Autodesk Inventor part; units mm, degrees
(part 2 of 2)
  line L452 (2.0688, 5.6455) -> (1.7172, 5.9716)
  line L453 (1.7172, 5.9716) -> (1.2814, 5.6264)
  line L454 (1.2814, 5.1401) -> (1.2814, 5.5243)
  line L455 (1.2814, 5.5243) -> (1.3618, 5.5243)
  line L456 (1.3618, 5.5243) -> (1.3618, 5.3813)
  line L457 (1.3618, 5.3813) -> (1.8895, 5.3813)
  line L458 (1.8895, 5.3813) -> (1.8895, 5.5243)
  line L459 (1.8895, 5.5243) -> (1.9616, 5.5243)
  spline S169 degree 2 poles (1.9616, 5.5243) (1.9616, 5.4432) (2.0075, 5.3667) (2.0713, 5.3616) knots 0 0 0 1 2 2 2
  line L460 (2.0713, 5.3616) -> (2.0713, 5.2799)
  line L461 (2.0713, 5.2799) -> (1.3618, 5.2799)
  line L462 (1.3618, 5.2799) -> (1.3618, 5.1401)
  line L463 (1.3618, 5.1401) -> (1.2814, 5.1401)
  line L464 (1.5519, 4.4887) -> (1.5519, 4.5825)
  line L465 (1.5519, 4.5825) -> (1.2814, 4.5825)
  line L466 (1.2814, 4.5825) -> (1.2814, 4.6839)
  line L467 (1.2814, 4.6839) -> (1.5519, 4.6839)
  line L468 (1.5519, 4.6839) -> (1.5519, 5.0317)
  line L469 (1.5519, 5.0317) -> (1.6629, 5.0317)
  line L470 (1.6629, 5.0317) -> (2.0688, 4.6794)
  line L471 (2.0688, 4.6794) -> (2.0688, 4.5825)
  line L472 (2.0688, 4.5825) -> (1.6368, 4.5825)
  line L473 (1.6368, 4.5825) -> (1.6368, 4.4887)
  line L474 (1.6368, 4.4887) -> (1.5519, 4.4887)
  line L475 (1.6368, 4.6839) -> (1.9443, 4.6839)
  line L476 (1.9443, 4.6839) -> (1.6368, 4.9487)
  line L477 (1.6368, 4.9487) -> (1.6368, 4.6839)
  point P0 (0, 0)
  dimension "d0" = 53.34
  dimension "d1" = 66.04
  dimension "d2" = 66.04
  dimension "d3" = 2.032
  dimension "d4" = 12.7
  dimension "d5" = 2.286
  dimension "d6" = 33.401
  dimension "d23" = 0.4572
  dimension "d24" = 1.651
  dimension "d25" = 0.4572
  dimension "d26" = 1.651
  dimension "d27" = 0.4572
  dimension "d28" = 0.4572
  dimension "d29" = 0.4572
  dimension "d30" = 0.6397
  dimension "d31" = 1.651
  constraints: 11 collinear, 9 coincident, 20 other
  measures "d23" distance between parallel lines of L35 L38
  measures "d24" distance between parallel lines of L36 L41
  measures "d25" distance between parallel lines of L0 L42
  measures "d26" distance between parallel lines of L13 L49
  measures "d27" distance between parallel lines of L16 L46
  measures "d28" distance between parallel lines of L66 L10
  measures "d29" distance between parallel lines of L6 L62
  measures "d30" distance between parallel lines of L2 L58
  measures "d31" distance between parallel lines of L29 L53
extrude "DET1" add sketch "Sketch3" along normal blind 0.254 contours S0 L78 L79 S1 S2 S3 S4 S5 S6 S7 S8 L80 L81 S9 S10 S11 S12 S13 S14 S15 | L82 L83 L84 L85 L86 L87 L88 L89 L90 L91 L92 L93 | L94 L95 L96 L97 L98 L99 S16 L100 L101 L102 L103 | L104 L105 L106 L107 L108 L109 L110 L111 L112 L113 L114 | S17 L118 L119 S18 S19 S20 S21 S22 S23 S24 S25 L120 L121 S26 S27 S28 S29 S30 S31 S32 | L122 L123 L124 L125 L126 L127 L128 L129 L130 L131 L132 L133 | L134 L135 L136 L137 L138 L139 S33 L140 L141 L142 L143 | L144 L145 L146 L147 L148 L149 L150 L151 L152 L153 L154 | S34 L158 L159 S35 S36 S37 S38 S39 S40 S41 S42 L160 L161 S43 S44 S45 S46 S47 S48 S49 | L162 L163 L164 L165 L166 L167 L168 L169 L170 L171 L172 L173 | L174 L175 L176 L177 L178 L179 S50 L180 L181 L182 L183 | L184 L185 L186 L187 L188 L189 L190 L191 L192 L193 L194 | S51 L198 L199 S52 S53 S54 S55 S56 S57 S58 S59 L200 L201 S60 S61 S62 S63 S64 S65 S66 | L202 L203 L204 L205 L206 L207 L208 L209 L210 L211 L212 L213 | L214 L215 L216 L217 L218 L219 S67 L220 L221 L222 L223 | L224 L225 L226 L227 L228 L229 L230 L231 L232 L233 L234 | S68 L238 L239 S69 S70 S71 S72 S73 S74 S75 S76 L240 L241 S77 S78 S79 S80 S81 S82 S83 | L242 L243 L244 L245 L246 L247 L248 L249 L250 L251 L252 L253 | L254 L255 L256 L257 L258 L259 S84 L260 L261 L262 L263 | L264 L265 L266 L267 L268 L269 L270 L271 L272 L273 L274 | S85 L278 L279 S86 S87 S88 S89 S90 S91 S92 S93 L280 L281 S94 S95 S96 S97 S98 S99 S100 | L282 L283 L284 L285 L286 L287 L288 L289 L290 L291 L292 L293 | L294 L295 L296 L297 L298 L299 S101 L300 L301 L302 L303 | L304 L305 L306 L307 L308 L309 L310 L311 L312 L313 L314 | S102 L318 L319 S103 S104 S105 S106 S107 S108 S109 S110 L320 L321 S111 S112 S113 S114 S115 S116 S117 | L322 L323 L324 L325 L326 L327 L328 L329 L330 L331 L332 L333 | L334 L335 L336 L337 L338 L339 S118 L340 L341 L342 L343 | L344 L345 L346 L347 L348 L349 L350 L351 L352 L353 L354 | S119 L358 L359 S120 S121 S122 S123 S124 S125 S126 S127 L360 L361 S128 S129 S130 S131 S132 S133 S134 | L362 L363 L364 L365 L366 L367 L368 L369 L370 L371 L372 L373 | L374 L375 L376 L377 L378 L379 S135 L380 L381 L382 L383 | L384 L385 L386 L387 L388 L389 L390 L391 L392 L393 L394 | S136 L398 L399 S137 S138 S139 S140 S141 S142 S143 S144 L400 L401 S145 S146 S147 S148 S149 S150 S151 | L402 L403 L404 L405 L406 L407 L408 L409 L410 L411 L412 L413 | L414 L415 L416 L417 L418 L419 S152 L420 L421 L422 L423 | L424 L425 L426 L427 L428 L429 L430 L431 L432 L433 L434 | S153 L438 L439 S154 S155 S156 S157 S158 S159 S160 S161 L440 L441 S162 S163 S164 S165 S166 S167 S168 | L442 L443 L444 L445 L446 L447 L448 L449 L450 L451 L452 L453 | L454 L455 L456 L457 L458 L459 S169 L460 L461 L462 L463 | L464 L465 L466 L467 L468 L469 L470 L471 L472 L473 L474
sketch "Sketch4" plane through (0, 1.524, 0) normal (0, 1, 0) x (1, 0, 0)
  line L0 (-26.67, 33.02) -> (-26.67, -33.02) projected
  line L1 (13.97, -33.02) -> (26.67, -33.02) projected
  line L2 (26.67, -33.02) -> (26.67, 33.02) projected
  line L3 (25.4, -31.75) -> (22.86, -31.75)
  line L4 (22.86, -31.75) -> (22.86, -11.43)
  line L5 (22.86, -11.43) -> (25.4, -11.43)
  line L6 (25.4, -11.43) -> (25.4, -31.75)
  line L7 (24.13, -31.75) -> (24.13, -11.43) construction
  line L8 (22.86, -10.287) -> (25.4, -10.287)
  line L9 (25.4, -10.287) -> (25.4, 15.113)
  line L10 (25.4, 15.113) -> (22.86, 15.113)
  line L11 (22.86, 15.113) -> (22.86, -10.287)
  line L12 (23.749, 14.224) -> (24.511, 14.224)
  line L13 (24.511, 14.224) -> (24.511, 13.462)
  line L14 (24.511, 13.462) -> (23.749, 13.462)
  line L15 (23.749, 13.462) -> (23.749, 14.224)
  line L16 (24.511, 13.462) -> (23.749, 14.224) construction
  line L17 (23.749, 13.462) -> (24.511, 14.224) construction
  line L18 (23.749, 11.684) -> (24.511, 11.684)
  line L19 (24.511, 11.684) -> (24.511, 10.922)
  line L20 (24.511, 10.922) -> (23.749, 10.922)
  line L21 (23.749, 10.922) -> (23.749, 11.684)
  line L22 (23.749, 9.144) -> (24.511, 9.144)
  line L23 (24.511, 9.144) -> (24.511, 8.382)
  line L24 (24.511, 8.382) -> (23.749, 8.382)
  line L25 (23.749, 8.382) -> (23.749, 9.144)
  line L26 (23.749, 6.604) -> (24.511, 6.604)
  line L27 (24.511, 6.604) -> (24.511, 5.842)
  line L28 (24.511, 5.842) -> (23.749, 5.842)
  line L29 (23.749, 5.842) -> (23.749, 6.604)
  line L30 (23.749, 4.064) -> (24.511, 4.064)
  line L31 (24.511, 4.064) -> (24.511, 3.302)
  line L32 (24.511, 3.302) -> (23.749, 3.302)
  line L33 (23.749, 3.302) -> (23.749, 4.064)
  line L34 (23.749, 1.524) -> (24.511, 1.524)
  line L35 (24.511, 1.524) -> (24.511, 0.762)
  line L36 (24.511, 0.762) -> (23.749, 0.762)
  line L37 (23.749, 0.762) -> (23.749, 1.524)
  line L38 (23.749, -1.016) -> (24.511, -1.016)
  line L39 (24.511, -1.016) -> (24.511, -1.778)
  line L40 (24.511, -1.778) -> (23.749, -1.778)
  line L41 (23.749, -1.778) -> (23.749, -1.016)
  line L42 (23.749, -3.556) -> (24.511, -3.556)
  line L43 (24.511, -3.556) -> (24.511, -4.318)
  line L44 (24.511, -4.318) -> (23.749, -4.318)
  line L45 (23.749, -4.318) -> (23.749, -3.556)
  line L46 (23.749, -6.096) -> (24.511, -6.096)
  line L47 (24.511, -6.096) -> (24.511, -6.858)
  line L48 (24.511, -6.858) -> (23.749, -6.858)
  line L49 (23.749, -6.858) -> (23.749, -6.096)
  line L50 (23.749, -8.636) -> (24.511, -8.636)
  line L51 (24.511, -8.636) -> (24.511, -9.398)
  line L52 (24.511, -9.398) -> (23.749, -9.398)
  line L53 (23.749, -9.398) -> (23.749, -8.636)
  line L54 (23.749, -12.319) -> (24.511, -12.319)
  line L55 (24.511, -12.319) -> (24.511, -13.081)
  line L56 (24.511, -13.081) -> (23.749, -13.081)
  line L57 (23.749, -13.081) -> (23.749, -12.319)
  line L58 (23.749, -12.319) -> (24.511, -13.081) construction
  line L59 (24.511, -12.319) -> (23.749, -13.081) construction
  line L60 (23.749, -14.859) -> (24.511, -14.859)
  line L61 (24.511, -14.859) -> (24.511, -15.621)
  line L62 (24.511, -15.621) -> (23.749, -15.621)
  line L63 (23.749, -15.621) -> (23.749, -14.859)
  line L64 (23.749, -17.399) -> (24.511, -17.399)
  line L65 (24.511, -17.399) -> (24.511, -18.161)
  line L66 (24.511, -18.161) -> (23.749, -18.161)
  line L67 (23.749, -18.161) -> (23.749, -17.399)
  line L68 (23.749, -19.939) -> (24.511, -19.939)
  line L69 (24.511, -19.939) -> (24.511, -20.701)
  line L70 (24.511, -20.701) -> (23.749, -20.701)
  line L71 (23.749, -20.701) -> (23.749, -19.939)
  line L72 (23.749, -22.479) -> (24.511, -22.479)
  line L73 (24.511, -22.479) -> (24.511, -23.241)
  line L74 (24.511, -23.241) -> (23.749, -23.241)
  line L75 (23.749, -23.241) -> (23.749, -22.479)
  line L76 (23.749, -25.019) -> (24.511, -25.019)
  line L77 (24.511, -25.019) -> (24.511, -25.781)
  line L78 (24.511, -25.781) -> (23.749, -25.781)
  line L79 (23.749, -25.781) -> (23.749, -25.019)
  line L80 (23.749, -27.559) -> (24.511, -27.559)
  line L81 (24.511, -27.559) -> (24.511, -28.321)
  line L82 (24.511, -28.321) -> (23.749, -28.321)
  line L83 (23.749, -28.321) -> (23.749, -27.559)
  line L84 (23.749, -30.099) -> (24.511, -30.099)
  line L85 (24.511, -30.099) -> (24.511, -30.861)
  line L86 (24.511, -30.861) -> (23.749, -30.861)
  line L87 (23.749, -30.861) -> (23.749, -30.099)
  line L88 (-21.59, -31.75) -> (-24.13, -31.75)
  line L89 (-24.13, -31.75) -> (-24.13, -16.51)
  line L90 (-24.13, -16.51) -> (-21.59, -16.51)
  line L91 (-21.59, -16.51) -> (-21.59, -31.75)
  line L92 (-22.479, -17.399) -> (-23.241, -17.399)
  line L93 (-23.241, -17.399) -> (-23.241, -18.161)
  line L94 (-23.241, -18.161) -> (-22.479, -18.161)
  line L95 (-22.479, -18.161) -> (-22.479, -17.399)
  line L96 (-22.479, -18.161) -> (-23.241, -17.399) construction
  line L97 (-22.479, -17.399) -> (-23.241, -18.161) construction
  line L98 (-22.479, -19.939) -> (-23.241, -19.939)
  line L99 (-23.241, -19.939) -> (-23.241, -20.701)
  line L100 (-23.241, -20.701) -> (-22.479, -20.701)
  line L101 (-22.479, -20.701) -> (-22.479, -19.939)
  line L102 (-22.479, -22.479) -> (-23.241, -22.479)
  line L103 (-23.241, -22.479) -> (-23.241, -23.241)
  line L104 (-23.241, -23.241) -> (-22.479, -23.241)
  line L105 (-22.479, -23.241) -> (-22.479, -22.479)
  line L106 (-22.479, -25.019) -> (-23.241, -25.019)
  line L107 (-23.241, -25.019) -> (-23.241, -25.781)
  line L108 (-23.241, -25.781) -> (-22.479, -25.781)
  line L109 (-22.479, -25.781) -> (-22.479, -25.019)
  line L110 (-22.479, -27.559) -> (-23.241, -27.559)
  line L111 (-23.241, -27.559) -> (-23.241, -28.321)
  line L112 (-23.241, -28.321) -> (-22.479, -28.321)
  line L113 (-22.479, -28.321) -> (-22.479, -27.559)
  line L114 (-22.479, -30.099) -> (-23.241, -30.099)
  line L115 (-23.241, -30.099) -> (-23.241, -30.861)
  line L116 (-23.241, -30.861) -> (-22.479, -30.861)
  line L117 (-22.479, -30.861) -> (-22.479, -30.099)
  line L118 (-24.13, -15.367) -> (-21.59, -15.367)
  line L119 (-21.59, -15.367) -> (-21.59, 4.953)
  line L120 (-21.59, 4.953) -> (-24.13, 4.953)
  line L121 (-24.13, 4.953) -> (-24.13, -15.367)
  line L122 (-23.241, 4.064) -> (-22.479, 4.064)
  line L123 (-22.479, 4.064) -> (-22.479, 3.302)
  line L124 (-22.479, 3.302) -> (-23.241, 3.302)
  line L125 (-23.241, 3.302) -> (-23.241, 4.064)
  line L126 (-23.241, 1.524) -> (-22.479, 1.524)
  line L127 (-22.479, 1.524) -> (-22.479, 0.762)
  line L128 (-22.479, 0.762) -> (-23.241, 0.762)
  line L129 (-23.241, 0.762) -> (-23.241, 1.524)
  line L130 (-23.241, -1.016) -> (-22.479, -1.016)
  line L131 (-22.479, -1.016) -> (-22.479, -1.778)
  line L132 (-22.479, -1.778) -> (-23.241, -1.778)
  line L133 (-23.241, -1.778) -> (-23.241, -1.016)
  line L134 (-23.241, -3.556) -> (-22.479, -3.556)
  line L135 (-22.479, -3.556) -> (-22.479, -4.318)
  line L136 (-22.479, -4.318) -> (-23.241, -4.318)
  line L137 (-23.241, -4.318) -> (-23.241, -3.556)
  line L138 (-23.241, -6.096) -> (-22.479, -6.096)
  line L139 (-22.479, -6.096) -> (-22.479, -6.858)
  line L140 (-22.479, -6.858) -> (-23.241, -6.858)
  line L141 (-23.241, -6.858) -> (-23.241, -6.096)
  line L142 (-23.241, -8.636) -> (-22.479, -8.636)
  line L143 (-22.479, -8.636) -> (-22.479, -9.398)
  line L144 (-22.479, -9.398) -> (-23.241, -9.398)
  line L145 (-23.241, -9.398) -> (-23.241, -8.636)
  line L146 (-23.241, -11.176) -> (-22.479, -11.176)
  line L147 (-22.479, -11.176) -> (-22.479, -11.938)
  line L148 (-22.479, -11.938) -> (-23.241, -11.938)
  line L149 (-23.241, -11.938) -> (-23.241, -11.176)
  line L150 (-23.241, -13.716) -> (-22.479, -13.716)
  line L151 (-22.479, -13.716) -> (-22.479, -14.478)
  line L152 (-22.479, -14.478) -> (-23.241, -14.478)
  line L153 (-23.241, -14.478) -> (-23.241, -13.716)
  point P0 (0, 0)
  point P1 (24.13, 13.843)
  point P2 (24.13, -12.7)
  point P3 (-22.86, -17.78)
  dimension "d34" = 2.54
  dimension "d36" = 20.32
  dimension "d37" = 1.27
  dimension "d38" = 1.27
  dimension "d39" = 25.4
  dimension "d40" = 1.143
  dimension "d42" = 0.762
  dimension "d44" = 1.27
  dimension "d46" = 1.27
  dimension "d49" = 2.54
  dimension "d54" = 1.27
  dimension "d57" = 2.54
  dimension "d62" = 0.889
  dimension "d63" = 0.889
  dimension "d64" = 2.54
  dimension "d65" = 15.24
  dimension "d66" = 0.762
  dimension "d68" = 0.889
  dimension "d69" = 1.27
  dimension "d72" = 2.54
  dimension "d77" = 20.32
  dimension "d78" = 1.143
  dimension "d79" = 0.762
  dimension "d81" = 0.889
  dimension "d84" = 2.54
  constraints: 302 end point, 16 parallel, 10 perpendicular, 8 horizontal, 7 equal length, 6 collinear, 5 midpoint, 4 vertical, 224 other
  measures "d34" distance between parallel lines of L6 L4
  measures "d36" distance of L5.end L3.start
  measures "d37" distance between parallel lines of L6 L2
  measures "d38" distance between parallel lines of L1 L3
  measures "d39" distance of L8.end L9.end
  measures "d40" distance between parallel lines of L5 L8
  measures "d42" distance of L12.end L13.end
  measures "d44" distance from line of L11 point (24.13, 13.843)
  measures "d46" distance from line of L10 point (24.13, 13.843)
  measures "d49" distance of L12.end L19.start
  measures "d54" distance from line of L5 point (24.13, -12.7)
  measures "d57" distance of L56.end L63.start
  measures "d62" distance between parallel lines of L3 L86
  measures "d63" distance between parallel lines of L8 L52
  measures "d64" distance between parallel lines of L0 L89
  measures "d65" distance of L88.end L89.end
  measures "d66" distance of L94.end L93.end
  measures "d68" distance between parallel lines of L89 L93
  measures "d69" distance from line of L90 point (-22.86, -17.78)
  measures "d72" distance of L94.end L101.start
  measures "d77" distance of L120.end L118.start
  measures "d78" distance between parallel lines of L90 L118
  measures "d79" distance of L122.start L122.end
  measures "d81" distance between parallel lines of L120 L122
  measures "d84" distance of L123.end L128.start
extrude "Extrusion4" add sketch "Sketch4" along normal blind 8.636
sketch "Sketch5" plane through (0, 1.524, 0) normal (0, 1, 0) x (1, 0, 0)
  line L0 (-22.479, 3.302) -> (-22.479, 4.064) projected
  line L1 (-22.479, 4.064) -> (-23.241, 4.064) projected
  line L2 (-23.241, 4.064) -> (-23.241, 3.302) projected
  line L3 (-23.241, 3.302) -> (-22.479, 3.302) projected
  line L4 (-23.241, 0.762) -> (-22.479, 0.762) projected
  line L5 (-22.479, 0.762) -> (-22.479, 1.524) projected
  line L6 (-22.479, 1.524) -> (-23.241, 1.524) projected
  line L7 (-23.241, 1.524) -> (-23.241, 0.762) projected
  line L8 (-23.241, -1.778) -> (-22.479, -1.778) projected
  line L9 (-22.479, -1.778) -> (-22.479, -1.016) projected
  line L10 (-22.479, -1.016) -> (-23.241, -1.016) projected
  line L11 (-23.241, -1.016) -> (-23.241, -1.778) projected
  line L12 (-23.241, -4.318) -> (-22.479, -4.318) projected
  line L13 (-22.479, -4.318) -> (-22.479, -3.556) projected
  line L14 (-22.479, -3.556) -> (-23.241, -3.556) projected
  line L15 (-23.241, -3.556) -> (-23.241, -4.318) projected
  line L16 (-23.241, -6.858) -> (-22.479, -6.858) projected
  line L17 (-22.479, -6.858) -> (-22.479, -6.096) projected
  line L18 (-22.479, -6.096) -> (-23.241, -6.096) projected
  line L19 (-23.241, -6.096) -> (-23.241, -6.858) projected
  line L20 (-23.241, -9.398) -> (-22.479, -9.398) projected
  line L21 (-22.479, -9.398) -> (-22.479, -8.636) projected
  line L22 (-22.479, -8.636) -> (-23.241, -8.636) projected
  line L23 (-23.241, -8.636) -> (-23.241, -9.398) projected
  line L24 (-23.241, -11.938) -> (-22.479, -11.938) projected
  line L25 (-22.479, -11.938) -> (-22.479, -11.176) projected
  line L26 (-22.479, -11.176) -> (-23.241, -11.176) projected
  line L27 (-23.241, -11.176) -> (-23.241, -11.938) projected
  line L28 (-23.241, -14.478) -> (-22.479, -14.478) projected
  line L29 (-22.479, -14.478) -> (-22.479, -13.716) projected
  line L30 (-22.479, -13.716) -> (-23.241, -13.716) projected
  line L31 (-23.241, -13.716) -> (-23.241, -14.478) projected
  line L32 (-22.479, -18.161) -> (-22.479, -17.399) projected
  line L33 (-22.479, -17.399) -> (-23.241, -17.399) projected
  line L34 (-23.241, -17.399) -> (-23.241, -18.161) projected
  line L35 (-23.241, -18.161) -> (-22.479, -18.161) projected
  line L36 (-23.241, -19.939) -> (-23.241, -20.701) projected
  line L37 (-23.241, -20.701) -> (-22.479, -20.701) projected
  line L38 (-22.479, -20.701) -> (-22.479, -19.939) projected
  line L39 (-22.479, -19.939) -> (-23.241, -19.939) projected
  line L40 (-23.241, -22.479) -> (-23.241, -23.241) projected
  line L41 (-23.241, -23.241) -> (-22.479, -23.241) projected
  line L42 (-22.479, -23.241) -> (-22.479, -22.479) projected
  line L43 (-22.479, -22.479) -> (-23.241, -22.479) projected
  line L44 (-23.241, -25.019) -> (-23.241, -25.781) projected
  line L45 (-23.241, -25.781) -> (-22.479, -25.781) projected
  line L46 (-22.479, -25.781) -> (-22.479, -25.019) projected
  line L47 (-22.479, -25.019) -> (-23.241, -25.019) projected
  line L48 (-23.241, -27.559) -> (-23.241, -28.321) projected
  line L49 (-23.241, -28.321) -> (-22.479, -28.321) projected
  line L50 (-22.479, -28.321) -> (-22.479, -27.559) projected
  line L51 (-22.479, -27.559) -> (-23.241, -27.559) projected
  line L52 (-23.241, -30.099) -> (-23.241, -30.861) projected
  line L53 (-23.241, -30.861) -> (-22.479, -30.861) projected
  line L54 (-22.479, -30.861) -> (-22.479, -30.099) projected
  line L55 (-22.479, -30.099) -> (-23.241, -30.099) projected
  line L56 (24.511, 13.462) -> (24.511, 14.224) projected
  line L57 (24.511, 14.224) -> (23.749, 14.224) projected
  line L58 (23.749, 14.224) -> (23.749, 13.462) projected
  line L59 (23.749, 13.462) -> (24.511, 13.462) projected
  line L60 (24.511, 10.922) -> (24.511, 11.684) projected
  line L61 (24.511, 11.684) -> (23.749, 11.684) projected
  line L62 (23.749, 11.684) -> (23.749, 10.922) projected
  line L63 (23.749, 10.922) -> (24.511, 10.922) projected
  line L64 (24.511, 8.382) -> (24.511, 9.144) projected
  line L65 (24.511, 9.144) -> (23.749, 9.144) projected
  line L66 (23.749, 9.144) -> (23.749, 8.382) projected
  line L67 (23.749, 8.382) -> (24.511, 8.382) projected
  line L68 (24.511, 5.842) -> (24.511, 6.604) projected
  line L69 (24.511, 6.604) -> (23.749, 6.604) projected
  line L70 (23.749, 6.604) -> (23.749, 5.842) projected
  line L71 (23.749, 5.842) -> (24.511, 5.842) projected
  line L72 (24.511, 3.302) -> (24.511, 4.064) projected
  line L73 (24.511, 4.064) -> (23.749, 4.064) projected
  line L74 (23.749, 4.064) -> (23.749, 3.302) projected
  line L75 (23.749, 3.302) -> (24.511, 3.302) projected
  line L76 (24.511, 0.762) -> (24.511, 1.524) projected
  line L77 (24.511, 1.524) -> (23.749, 1.524) projected
  line L78 (23.749, 1.524) -> (23.749, 0.762) projected
  line L79 (23.749, 0.762) -> (24.511, 0.762) projected
  line L80 (24.511, -1.778) -> (24.511, -1.016) projected
  line L81 (24.511, -1.016) -> (23.749, -1.016) projected
  line L82 (23.749, -1.016) -> (23.749, -1.778) projected
  line L83 (23.749, -1.778) -> (24.511, -1.778) projected
  line L84 (24.511, -4.318) -> (24.511, -3.556) projected
  line L85 (24.511, -3.556) -> (23.749, -3.556) projected
  line L86 (23.749, -3.556) -> (23.749, -4.318) projected
  line L87 (23.749, -4.318) -> (24.511, -4.318) projected
  line L88 (24.511, -6.858) -> (24.511, -6.096) projected
  line L89 (24.511, -6.096) -> (23.749, -6.096) projected
  line L90 (23.749, -6.096) -> (23.749, -6.858) projected
  line L91 (23.749, -6.858) -> (24.511, -6.858) projected
  line L92 (24.511, -9.398) -> (24.511, -8.636) projected
  line L93 (24.511, -8.636) -> (23.749, -8.636) projected
  line L94 (23.749, -8.636) -> (23.749, -9.398) projected
  line L95 (23.749, -9.398) -> (24.511, -9.398) projected
  line L96 (24.511, -13.081) -> (24.511, -12.319) projected
  line L97 (24.511, -12.319) -> (23.749, -12.319) projected
  line L98 (23.749, -12.319) -> (23.749, -13.081) projected
  line L99 (23.749, -13.081) -> (24.511, -13.081) projected
  line L100 (23.749, -14.859) -> (23.749, -15.621) projected
  line L101 (23.749, -15.621) -> (24.511, -15.621) projected
  line L102 (24.511, -15.621) -> (24.511, -14.859) projected
  line L103 (24.511, -14.859) -> (23.749, -14.859) projected
  line L104 (23.749, -17.399) -> (23.749, -18.161) projected
  line L105 (23.749, -18.161) -> (24.511, -18.161) projected
  line L106 (24.511, -18.161) -> (24.511, -17.399) projected
  line L107 (24.511, -17.399) -> (23.749, -17.399) projected
  line L108 (23.749, -19.939) -> (23.749, -20.701) projected
  line L109 (23.749, -20.701) -> (24.511, -20.701) projected
  line L110 (24.511, -20.701) -> (24.511, -19.939) projected
  line L111 (24.511, -19.939) -> (23.749, -19.939) projected
  line L112 (23.749, -22.479) -> (23.749, -23.241) projected
  line L113 (23.749, -23.241) -> (24.511, -23.241) projected
  line L114 (24.511, -23.241) -> (24.511, -22.479) projected
  line L115 (24.511, -22.479) -> (23.749, -22.479) projected
  line L116 (23.749, -25.019) -> (23.749, -25.781) projected
  line L117 (23.749, -25.781) -> (24.511, -25.781) projected
  line L118 (24.511, -25.781) -> (24.511, -25.019) projected
  line L119 (24.511, -25.019) -> (23.749, -25.019) projected
  line L120 (23.749, -27.559) -> (23.749, -28.321) projected
  line L121 (23.749, -28.321) -> (24.511, -28.321) projected
  line L122 (24.511, -28.321) -> (24.511, -27.559) projected
  line L123 (24.511, -27.559) -> (23.749, -27.559) projected
  line L124 (23.749, -30.099) -> (23.749, -30.861) projected
  line L125 (23.749, -30.861) -> (24.511, -30.861) projected
  line L126 (24.511, -30.861) -> (24.511, -30.099) projected
  line L127 (24.511, -30.099) -> (23.749, -30.099) projected
  point P0 (0, 0)
extrude "Extrusion5" add sketch "Sketch5" against normal blind 14.605
fillet "Fillet1" radius 0.3969 128 edges at (-22.86, 0, 30.861) (-22.479, 0, 30.48) (-22.86, 0, 30.099) (-23.241, 0, 30.48) (-22.86, 0, 28.321) (-22.479, 0, 27.94) (-22.86, 0, 27.559) (-23.241, 0, 27.94) (-22.86, 0, 25.781) (-22.479, 0, 25.4) (-22.86, 0, 25.019) (-23.241, 0, 25.4) (-22.86, 0, 23.241) (-22.479, 0, 22.86) (-22.86, 0, 22.479) (-23.241, 0, 22.86) (-22.86, 0, 20.701) (-22.479, 0, 20.32) (-22.86, 0, 19.939) (-23.241, 0, 20.32) (-22.86, 0, 17.399) (-23.241, 0, 17.78) (-22.86, 0, 18.161) (-22.479, 0, 17.78) (-22.479, 0, 14.097) (-22.86, 0, 13.716) (-23.241, 0, 14.097) (-22.86, 0, 14.478) (-22.479, 0, 11.557) (-22.86, 0, 11.176) (-23.241, 0, 11.557) (-22.86, 0, 11.938) (-22.479, 0, 9.017) (-22.86, 0, 8.636) (-23.241, 0, 9.017) (-22.86, 0, 9.398) (-22.479, 0, 6.477) (-22.86, 0, 6.096) (-23.241, 0, 6.477) (-22.86, 0, 6.858) (-22.86, 0, 3.556) (-23.241, 0, 3.937) (-22.86, 0, 4.318) (-22.479, 0, 3.937) (-22.479, 0, 1.397) (-22.86, 0, 1.016) (-23.241, 0, 1.397) (-22.86, 0, 1.778) (-22.479, 0, -1.143) (-22.86, 0, -1.524) (-23.241, 0, -1.143) (-22.86, 0, -0.762) (-22.86, 0, -4.064) (-23.241, 0, -3.683) (-22.86, 0, -3.302) (-22.479, 0, -3.683) (24.13, 0, 30.861) (24.511, 0, 30.48) (24.13, 0, 30.099) (23.749, 0, 30.48) (24.13, 0, 28.321) (24.511, 0, 27.94) (24.13, 0, 27.559) (23.749, 0, 27.94) (24.13, 0, 25.781) (24.511, 0, 25.4) (24.13, 0, 25.019) (23.749, 0, 25.4) (24.13, 0, 23.241) (24.511, 0, 22.86) (24.13, 0, 22.479) (23.749, 0, 22.86) (24.13, 0, 20.701) (24.511, 0, 20.32) (24.13, 0, 19.939) (23.749, 0, 20.32) (24.13, 0, 18.161) (24.511, 0, 17.78) (24.13, 0, 17.399) (23.749, 0, 17.78) (24.13, 0, 15.621) (24.511, 0, 15.24) (24.13, 0, 14.859) (23.749, 0, 15.24) (24.13, 0, 12.319) (23.749, 0, 12.7) (24.13, 0, 13.081) (24.511, 0, 12.7) (24.13, 0, 8.636) (23.749, 0, 9.017) (24.13, 0, 9.398) (24.511, 0, 9.017) (24.13, 0, 6.096) (23.749, 0, 6.477) (24.13, 0, 6.858) (24.511, 0, 6.477) (24.13, 0, 3.556) (23.749, 0, 3.937) (24.13, 0, 4.318) (24.511, 0, 3.937) (24.13, 0, 1.016) (23.749, 0, 1.397) (24.13, 0, 1.778) (24.511, 0, 1.397) (24.13, 0, -1.524) (23.749, 0, -1.143) (24.13, 0, -0.762) (24.511, 0, -1.143) (24.13, 0, -4.064) (23.749, 0, -3.683) (24.13, 0, -3.302) (24.511, 0, -3.683) (24.13, 0, -6.604) (23.749, 0, -6.223) (24.13, 0, -5.842) (24.511, 0, -6.223) (24.13, 0, -9.144) (23.749, 0, -8.763) (24.13, 0, -8.382) (24.511, 0, -8.763) (24.13, 0, -11.684) (23.749, 0, -11.303) (24.13, 0, -10.922) (24.511, 0, -11.303) (24.13, 0, -14.224) (23.749, 0, -13.843) (24.13, 0, -13.462) (24.511, 0, -13.843)
chamfer "Chamfer1" distance 0.1905 angle 45 71 edges at (24.511, -13.081, 30.48) (24.13, -13.081, 30.861) (23.749, -13.081, 30.48) (24.13, -13.081, 30.099) (24.511, -13.081, 27.94) (24.13, -13.081, 28.321) (23.749, -13.081, 27.94) (24.13, -13.081, 27.559) (24.13, -13.081, 25.781) (24.511, -13.081, 25.4) (24.13, -13.081, 25.019) (23.749, -13.081, 25.4) (24.511, -13.081, 22.86) (24.13, -13.081, 22.479) (23.749, -13.081, 22.86) (24.13, -13.081, 20.701) (24.511, -13.081, 20.32) (23.749, -13.081, 20.32) (24.13, -13.081, 19.939) (24.13, -13.081, 18.161) (24.511, -13.081, 17.78) (23.749, -13.081, 17.78) (24.13, -13.081, 17.399) (24.511, -13.081, 15.24) (24.13, -13.081, 15.621) (23.749, -13.081, 15.24) (24.13, -13.081, 14.859) (24.13, -13.081, 13.081) (24.511, -13.081, 12.7) (23.749, -13.081, 12.7) (24.13, -13.081, 12.319) (24.13, -13.081, 9.398) (24.511, -13.081, 9.017) (24.13, -13.081, 8.636) (23.749, -13.081, 9.017) (24.13, -13.081, 6.858) (24.511, -13.081, 6.477) (23.749, -13.081, 6.477) (24.13, -13.081, 6.096) (24.13, -13.081, 4.318) (24.511, -13.081, 3.937) (23.749, -13.081, 3.937) (24.13, -13.081, 3.556) (24.13, -13.081, 1.778) (24.511, -13.081, 1.397) (23.749, -13.081, 1.397) (24.13, -13.081, 1.016) (24.13, -13.081, -0.762) (24.511, -13.081, -1.143) (24.13, -13.081, -1.524) (23.749, -13.081, -1.143) (24.13, -13.081, -3.302) (24.511, -13.081, -3.683) (23.749, -13.081, -3.683) (24.13, -13.081, -4.064) (24.13, -13.081, -5.842) (24.511, -13.081, -6.223) (23.749, -13.081, -6.223) (24.13, -13.081, -6.604) (24.13, -13.081, -8.382) (24.511, -13.081, -8.763) (23.749, -13.081, -8.763) (24.13, -13.081, -9.144) (24.511, -13.081, -11.303) (24.13, -13.081, -10.922) (24.13, -13.081, -11.684) (23.749, -13.081, -11.303) (24.511, -13.081, -13.843) (24.13, -13.081, -13.462) (23.749, -13.081, -13.843) (24.13, -13.081, -14.224)
sketch "Sketch6" plane through (0, 1.524, 0) normal (0, 1, 0) x (1, 0, 0)
  line L0 (22.86, -31.75) -> (22.86, -11.43) projected
  line L1 (13.97, -33.02) -> (26.67, -33.02) projected
  line L2 (26.67, -33.02) -> (26.67, 33.02) projected
  line L3 (7.747, -27.94) -> (15.367, -27.94)
  line L4 (15.367, -27.94) -> (15.367, -22.225)
  line L5 (15.367, -22.225) -> (7.747, -22.225)
  line L6 (7.747, -22.225) -> (7.747, -27.94)
  line L7 (9.1186, -27.94) -> (13.9954, -27.94)
  line L8 (13.9954, -27.94) -> (13.9954, -27.051)
  line L9 (13.9954, -27.051) -> (9.1186, -27.051)
  line L10 (9.1186, -27.051) -> (9.1186, -27.94)
  line L11 (7.747, -20.3962) -> (15.367, -20.3962)
  line L12 (15.367, -20.3962) -> (15.367, -14.6812)
  line L13 (15.367, -14.6812) -> (7.747, -14.6812)
  line L14 (7.747, -14.6812) -> (7.747, -20.3962)
  line L15 (9.1186, -20.3962) -> (13.9954, -20.3962)
  line L16 (13.9954, -20.3962) -> (13.9954, -19.5072)
  line L17 (13.9954, -19.5072) -> (9.1186, -19.5072)
  line L18 (9.1186, -19.5072) -> (9.1186, -20.3962)
  line L19 (7.747, -12.8524) -> (15.367, -12.8524)
  line L20 (15.367, -12.8524) -> (15.367, -7.1374)
  line L21 (15.367, -7.1374) -> (7.747, -7.1374)
  line L22 (7.747, -7.1374) -> (7.747, -12.8524)
  line L23 (9.1186, -12.8524) -> (13.9954, -12.8524)
  line L24 (13.9954, -12.8524) -> (13.9954, -11.9634)
  line L25 (13.9954, -11.9634) -> (9.1186, -11.9634)
  line L26 (9.1186, -11.9634) -> (9.1186, -12.8524)
  line L27 (7.747, -5.3086) -> (15.367, -5.3086)
  line L28 (15.367, -5.3086) -> (15.367, 0.4064)
  line L29 (15.367, 0.4064) -> (7.747, 0.4064)
  line L30 (7.747, 0.4064) -> (7.747, -5.3086)
  line L31 (9.1186, -5.3086) -> (13.9954, -5.3086)
  line L32 (13.9954, -5.3086) -> (13.9954, -4.4196)
  line L33 (13.9954, -4.4196) -> (9.1186, -4.4196)
  line L34 (9.1186, -4.4196) -> (9.1186, -5.3086)
  line L35 (6.477, 7.8994) -> (16.637, 7.8994)
  line L36 (16.637, 7.8994) -> (16.637, 2.1844)
  line L37 (16.637, 2.1844) -> (6.477, 2.1844)
  line L38 (6.477, 2.1844) -> (6.477, 7.8994)
  line L39 (7.8105, 2.1844) -> (15.3035, 2.1844)
  line L40 (15.3035, 2.1844) -> (15.3035, 3.0734)
  line L41 (15.3035, 3.0734) -> (7.8105, 3.0734)
  line L42 (7.8105, 3.0734) -> (7.8105, 2.1844)
  line L43 (6.477, 15.5194) -> (16.637, 15.5194)
  line L44 (16.637, 15.5194) -> (16.637, 9.8044)
  line L45 (16.637, 9.8044) -> (6.477, 9.8044)
  line L46 (6.477, 9.8044) -> (6.477, 15.5194)
  line L47 (7.8105, 9.8044) -> (15.3035, 9.8044)
  line L48 (15.3035, 9.8044) -> (15.3035, 10.6934)
  line L49 (15.3035, 10.6934) -> (7.8105, 10.6934)
  line L50 (7.8105, 10.6934) -> (7.8105, 9.8044)
  line L51 (8.636, -25.0698) -> (9.271, -25.0698)
  line L52 (9.271, -25.0698) -> (9.271, -25.7048)
  line L53 (9.271, -25.7048) -> (8.636, -25.7048)
  line L54 (8.636, -25.7048) -> (8.636, -25.0698)
  line L55 (11.557, -28.1305) -> (11.557, -31.9941) construction
  line L56 (14.478, -25.0698) -> (13.843, -25.0698)
  line L57 (13.843, -25.0698) -> (13.843, -25.7048)
  line L58 (13.843, -25.7048) -> (14.478, -25.7048)
  line L59 (14.478, -25.7048) -> (14.478, -25.0698)
  line L60 (11.2395, -25.0698) -> (11.8745, -25.0698)
  line L61 (11.8745, -25.0698) -> (11.8745, -25.7048)
  line L62 (11.8745, -25.7048) -> (11.2395, -25.7048)
  line L63 (11.2395, -25.7048) -> (11.2395, -25.0698)
  line L64 (11.2395, -25.0698) -> (11.8745, -25.7048) construction
  line L65 (11.8745, -25.0698) -> (11.2395, -25.7048) construction
  line L66 (8.636, -17.526) -> (9.271, -17.526)
  line L67 (9.271, -17.526) -> (9.271, -18.161)
  line L68 (9.271, -18.161) -> (8.636, -18.161)
  line L69 (8.636, -18.161) -> (8.636, -17.526)
  line L70 (14.478, -18.161) -> (14.478, -17.526)
  line L71 (14.478, -17.526) -> (13.843, -17.526)
  line L72 (13.843, -17.526) -> (13.843, -18.161)
  line L73 (13.843, -18.161) -> (14.478, -18.161)
  line L74 (11.2395, -17.526) -> (11.8745, -17.526)
  line L75 (11.8745, -17.526) -> (11.8745, -18.161)
  line L76 (11.8745, -18.161) -> (11.2395, -18.161)
  line L77 (11.2395, -18.161) -> (11.2395, -17.526)
  line L78 (8.636, -9.9822) -> (9.271, -9.9822)
  line L79 (9.271, -9.9822) -> (9.271, -10.6172)
  line L80 (9.271, -10.6172) -> (8.636, -10.6172)
  line L81 (8.636, -10.6172) -> (8.636, -9.9822)
  line L82 (14.478, -10.6172) -> (14.478, -9.9822)
  line L83 (14.478, -9.9822) -> (13.843, -9.9822)
  line L84 (13.843, -9.9822) -> (13.843, -10.6172)
  line L85 (13.843, -10.6172) -> (14.478, -10.6172)
  line L86 (11.2395, -9.9822) -> (11.8745, -9.9822)
  line L87 (11.8745, -9.9822) -> (11.8745, -10.6172)
  line L88 (11.8745, -10.6172) -> (11.2395, -10.6172)
  line L89 (11.2395, -10.6172) -> (11.2395, -9.9822)
  line L90 (8.636, -2.4384) -> (9.271, -2.4384)
  line L91 (9.271, -2.4384) -> (9.271, -3.0734)
  line L92 (9.271, -3.0734) -> (8.636, -3.0734)
  line L93 (8.636, -3.0734) -> (8.636, -2.4384)
  line L94 (14.478, -3.0734) -> (14.478, -2.4384)
  line L95 (14.478, -2.4384) -> (13.843, -2.4384)
  line L96 (13.843, -2.4384) -> (13.843, -3.0734)
  line L97 (13.843, -3.0734) -> (14.478, -3.0734)
  line L98 (11.2395, -2.4384) -> (11.8745, -2.4384)
  line L99 (11.8745, -2.4384) -> (11.8745, -3.0734)
  line L100 (11.8745, -3.0734) -> (11.2395, -3.0734)
  line L101 (11.2395, -3.0734) -> (11.2395, -2.4384)
  line L102 (7.366, 5.0546) -> (8.001, 5.0546)
  line L103 (8.001, 5.0546) -> (8.001, 4.4196)
  line L104 (8.001, 4.4196) -> (7.366, 4.4196)
  line L105 (7.366, 4.4196) -> (7.366, 5.0546)
  line L106 (9.9441, 4.4196) -> (10.5791, 4.4196)
  line L107 (10.5791, 4.4196) -> (10.5791, 5.0546)
  line L108 (10.5791, 5.0546) -> (9.9441, 5.0546)
  line L109 (9.9441, 5.0546) -> (9.9441, 4.4196)
  line L110 (12.5349, 4.4196) -> (13.1699, 4.4196)
  line L111 (13.1699, 4.4196) -> (13.1699, 5.0546)
  line L112 (13.1699, 5.0546) -> (12.5349, 5.0546)
  line L113 (12.5349, 5.0546) -> (12.5349, 4.4196)
  line L114 (15.113, 4.4196) -> (15.748, 4.4196)
  line L115 (15.748, 4.4196) -> (15.748, 5.0546)
  line L116 (15.748, 5.0546) -> (15.113, 5.0546)
  line L117 (15.113, 5.0546) -> (15.113, 4.4196)
  line L118 (7.366, 12.5984) -> (8.001, 12.5984)
  line L119 (8.001, 12.5984) -> (8.001, 11.9634)
  line L120 (8.001, 11.9634) -> (7.366, 11.9634)
  line L121 (7.366, 11.9634) -> (7.366, 12.5984)
  line L122 (9.9441, 11.9634) -> (10.5791, 11.9634)
  line L123 (10.5791, 11.9634) -> (10.5791, 12.5984)
  line L124 (10.5791, 12.5984) -> (9.9441, 12.5984)
  line L125 (9.9441, 12.5984) -> (9.9441, 11.9634)
  line L126 (12.5349, 11.9634) -> (13.1699, 11.9634)
  line L127 (13.1699, 11.9634) -> (13.1699, 12.5984)
  line L128 (13.1699, 12.5984) -> (12.5349, 12.5984)
  line L129 (12.5349, 12.5984) -> (12.5349, 11.9634)
  line L130 (15.113, 11.9634) -> (15.748, 11.9634)
  line L131 (15.748, 11.9634) -> (15.748, 12.5984)
  line L132 (15.748, 12.5984) -> (15.113, 12.5984)
  line L133 (15.113, 12.5984) -> (15.113, 11.9634)
  point P0 (0, 0)
  point P1 (11.557, -25.3873)
  dimension "d97" = 5.715
  dimension "d99" = 7.62
  dimension "d100" = 5.08
  dimension "d101" = 7.493
  dimension "d102" = 4.8768
  dimension "d103" = 1.3716
  dimension "d104" = 0.889
  dimension "d107" = 7.5438
  dimension "d112" = 10.16
  dimension "d113" = 1.27
  dimension "d116" = 1.778
  dimension "d117" = 5.715
  dimension "d118" = 7.493
  dimension "d119" = 0.889
  dimension "d120" = 1.3335
  dimension "d123" = 7.62
  dimension "d128" = 0.635
  dimension "d129" = 0.889
  dimension "d130" = 2.8702
  dimension "d131" = 3.81
  dimension "d132" = 3.81
  dimension "d135" = 7.5438
  dimension "d141" = 0.889
  dimension "d142" = 2.8702
  dimension "d143" = 0.889
  dimension "d146" = 1.9431
  dimension "d147" = 1.9431
  dimension "d148" = 1.9558
  dimension "d151" = 7.5438
  constraints: 262 end point, 21 parallel, 11 equal length, 11 perpendicular, 10 horizontal, 6 point on line, 4 collinear, 4 symmetric about line, 4 vertical, 1 midpoint, 168 other
  measures "d97" distance of L5.end L3.start
  measures "d99" distance of L3.start L3.end
  measures "d100" distance between parallel lines of L3 L1
  measures "d101" distance between parallel lines of L0 L4
  measures "d102" distance of L8.end L9.end
  measures "d103" distance between parallel lines of L6 L10
  measures "d104" distance of L9.end L7.start
  measures "d107" distance of L5.end L14.start
  measures "d112" distance of L35.start L35.end
  measures "d113" distance between parallel lines of L38 L30
  measures "d116" distance between parallel lines of L29 L37
  measures "d117" distance of L35.end L36.end
  measures "d118" distance of L39.start L39.end
  measures "d119" distance of L39.end L40.end
  measures "d120" distance between parallel lines of L38 L42
  measures "d123" distance of L37.end L46.start
  measures "d128" distance of L52.end L53.end
  measures "d129" distance between parallel lines of L6 L54
  measures "d130" distance between parallel lines of L3 L51
  measures "d131" distance between parallel lines of L4 L55
  measures "d132" distance from line of L6 point (11.557, -25.387)
  measures "d135" distance of L51.end L67.start
  measures "d141" distance between parallel lines of L38 L105
  measures "d142" distance between parallel lines of L37 L102
  measures "d143" distance between parallel lines of L36 L115
  measures "d146" distance between parallel lines of L109 L103
  measures "d147" distance between parallel lines of L117 L111
  measures "d148" distance between parallel lines of L113 L107
  measures "d151" distance of L102.end L119.start
extrude "Extrusion6" add sketch "Sketch6" along normal blind 1.27 contours L6 L5 L4 L3 L8 L9 L10 | L14 L13 L12 L11 L16 L17 L18 | L22 L21 L20 L19 L24 L25 L26 | L30 L29 L28 L27 L32 L33 L34 | L35 L36 L37 L40 L41 L42 L38 | L43 L44 L45 L48 L49 L50 L46
extrude "Extrusion7" add sketch "Sketch6" along normal blind 11.5824 contours L10 L9 L8 L3 | L18 L17 L16 L11 | L26 L25 L24 L19 | L34 L33 L32 L27 | L42 L41 L40 L37 | L50 L49 L48 L45
extrude "Extrusion8" add sketch "Sketch6" along normal blind 11.176 contours L51 L52 L53 L54 | L59 L58 L57 L56 | L60 L61 L62 L63 | L66 L67 L68 L69 | L73 L72 L71 L70 | L74 L75 L76 L77 | L78 L79 L80 L81 | L85 L84 L83 L82 | L86 L87 L88 L89 | L90 L91 L92 L93 | L97 L96 L95 L94 | L98 L99 L100 L101 | L102 L103 L104 L105 | L109 L108 L107 L106 | L113 L112 L111 L110 | L117 L116 L115 L114 | L118 L119 L120 L121 | L125 L124 L123 L122 | L129 L128 L127 L126 | L133 L132 L131 L130
sketch "Sketch7" plane through (0, 1.524, 0) normal (0, 1, 0) x (1, 0, 0)
  line L0 (-26.67, 33.02) -> (-26.67, -33.02) projected
  line L1 (-22.0345, -35.306) -> (11.3665, -35.306) projected
  line L2 (-20.828, 5.2832) -> (-17.399, 5.2832)
  line L3 (-17.399, 5.2832) -> (-17.399, 2.794)
  line L4 (-17.399, 2.794) -> (-20.828, 2.794)
  line L5 (-20.828, 2.794) -> (-20.828, 5.2832)
  line L6 (-20.828, 8.5852) -> (-17.399, 8.5852)
  line L7 (-17.399, 8.5852) -> (-17.399, 6.096)
  line L8 (-17.399, 6.096) -> (-20.828, 6.096)
  line L9 (-20.828, 6.096) -> (-20.828, 8.5852)
  line L10 (-20.828, 11.8872) -> (-17.399, 11.8872)
  line L11 (-17.399, 11.8872) -> (-17.399, 9.398)
  line L12 (-17.399, 9.398) -> (-20.828, 9.398)
  line L13 (-20.828, 9.398) -> (-20.828, 11.8872)
  line L14 (-20.828, 15.1892) -> (-17.399, 15.1892)
  line L15 (-17.399, 15.1892) -> (-17.399, 12.7)
  line L16 (-17.399, 12.7) -> (-20.828, 12.7)
  line L17 (-20.828, 12.7) -> (-20.828, 15.1892)
  point P0 (0, 0)
  dimension "d162" = 3.429
  dimension "d163" = 2.4892
  dimension "d164" = 5.842
  dimension "d166" = 38.1
  dimension "d169" = 3.302
  constraints: 32 end point, 2 parallel, 1 horizontal, 1 perpendicular, 1 vertical, 24 other
  measures "d162" distance of L3.end L4.end
  measures "d163" distance of L2.end L3.end
  measures "d164" distance between parallel lines of L0 L5
  measures "d166" distance between parallel lines of L1 L4
  measures "d169" distance of L4.end L9.start
extrude "Extrusion9" add sketch "Sketch7" along normal blind 1.905
fillet "Fillet2" radius 0.3969 32 edges at (-19.1135, 3.429, -5.2832) (-20.828, 3.429, -4.0386) (-19.1135, 3.429, -2.794) (-17.399, 3.429, -4.0386) (-19.1135, 3.429, -6.096) (-17.399, 3.429, -7.3406) (-19.1135, 3.429, -8.5852) (-20.828, 3.429, -7.3406) (-19.1135, 3.429, -12.7) (-17.399, 3.429, -13.9446) (-19.1135, 3.429, -15.1892) (-20.828, 3.429, -13.9446) (-19.1135, 3.429, -9.398) (-17.399, 3.429, -10.6426) (-19.1135, 3.429, -11.8872) (-20.828, 3.429, -10.6426) (-17.399, 2.4765, -5.2832) (-17.399, 2.4765, -2.794) (-20.828, 2.4765, -2.794) (-20.828, 2.4765, -5.2832) (-20.828, 2.4765, -6.096) (-20.828, 2.4765, -8.5852) (-17.399, 2.4765, -6.096) (-17.399, 2.4765, -8.5852) (-17.399, 2.4765, -9.398) (-20.828, 2.4765, -9.398) (-17.399, 2.4765, -11.8872) (-20.828, 2.4765, -11.8872) (-20.828, 2.4765, -12.7) (-17.399, 2.4765, -12.7) (-20.828, 2.4765, -15.1892) (-17.399, 2.4765, -15.1892)
sketch "Sketch8" plane through (0, 1.524, 0) normal (0, 1, 0) x (1, 0, 0)
  line L0 (26.67, 33.02) -> (-26.67, 33.02) projected
  line L1 (26.67, -33.02) -> (26.67, 33.02) projected
  line L2 (20.066, 23.495) -> (26.416, 23.495)
  line L3 (26.416, 23.495) -> (26.416, 29.845)
  line L4 (26.416, 29.845) -> (20.066, 29.845)
  line L5 (20.066, 29.845) -> (20.066, 23.495)
  point P0 (0, 0)
  dimension "d177" = 6.35
  dimension "d178" = 6.35
  dimension "d179" = 3.175
  dimension "d180" = 0.254
  constraints: 8 end point, 2 parallel, 1 horizontal, 1 perpendicular
  measures "d177" distance of L4.end L3.end
  measures "d178" distance of L3.end L2.end
  measures "d179" distance between parallel lines of L0 L4
  measures "d180" distance between parallel lines of L1 L3
extrude "Extrusion10" add sketch "Sketch8" along normal blind 2.4511
sketch "Sketch9" plane through (0, 3.9751, 0) normal (0, 1, 0) x (1, 0, 0)
  line L0 (20.066, 29.845) -> (26.416, 23.495) construction
  line L1 (26.416, 29.845) -> (20.066, 23.495) construction
  circle A0 centre (23.241, 26.67) radius 1.524
  point P0 (0, 0)
  dimension "d183" = 3.048
  constraints: 4 end point, 1 centre point, 1 midpoint, 1 perpendicular
  measures "d183" diameter of A0
extrude "Extrusion11" add sketch "Sketch9" along normal blind 1.143
sketch "Sketch10" plane through (0, 1.524, 0) normal (0, 1, 0) x (1, 0, 0)
  line L0 (-26.67, 33.02) -> (-26.67, -33.02) projected
  line L1 (-22.0345, -35.306) -> (11.3665, -35.306) projected
  line L2 (-9.0678, -23.1394) -> (-6.223, -23.1394)
  line L3 (-6.223, -23.1394) -> (-6.223, -20.066)
  line L4 (-6.223, -20.066) -> (-9.0678, -20.066)
  line L5 (-9.0678, -20.066) -> (-9.0678, -23.1394)
  line L6 (-0.635, -17.0942) -> (3.175, -17.0942)
  line L7 (3.175, -17.0942) -> (3.175, -25.6794)
  line L8 (3.175, -25.6794) -> (-0.635, -25.6794)
  line L9 (-0.635, -25.6794) -> (-0.635, -17.0942)
  line L10 (-11.4808, 3.1242) -> (-0.635, 3.1242)
  line L11 (-0.635, 3.1242) -> (-0.635, -12.6492)
  line L12 (-0.635, -12.6492) -> (-11.4808, -12.6492)
  line L13 (-11.4808, -12.6492) -> (-11.4808, 3.1242)
  point P0 (0, 0)
  dimension "d186" = 3.0734
  dimension "d188" = 2.8448
  dimension "d189" = 15.24
  dimension "d190" = 20.447
  dimension "d191" = 9.6266
  dimension "d192" = 8.5852
  dimension "d193" = 3.81
  dimension "d194" = 29.845
  dimension "d195" = 15.7734
  dimension "d196" = 10.8458
  dimension "d197" = 22.6568
  dimension "d198" = 26.035
  constraints: 24 end point, 6 parallel, 3 horizontal, 3 perpendicular
  measures "d186" distance of L4.end L2.start
  measures "d188" distance of L3.end L4.end
  measures "d189" distance between parallel lines of L1 L4
  measures "d190" distance between parallel lines of L0 L3
  measures "d191" distance between parallel lines of L1 L8
  measures "d192" distance of L6.end L7.end
  measures "d193" distance of L6.start L6.end
  measures "d194" distance between parallel lines of L0 L7
  measures "d195" distance of L12.end L10.start
  measures "d196" distance of L10.start L10.end
  measures "d197" distance between parallel lines of L1 L12
  measures "d198" distance between parallel lines of L0 L11
extrude "Extrusion12" add sketch "Sketch10" along normal blind 3.556 contours L10 L11 L12 L13
extrude "Extrusion13" add sketch "Sketch10" along normal blind 1.7526 contours L6 L7 L8 L9
extrude "Extrusion14" add sketch "Sketch10" along normal blind 0.9906 contours L5 L4 L3 L2
equation "\"d17\" = d14"
equation "\"d18\" = d17"
equation "\"d19\" = d17"
equation "\"d25\" = d23"
equation "\"d26\" = d24"
equation "\"d27\" = d23"
equation "\"d28\" = d27"
equation "\"d29\" = d28"
equation "\"d31\" = d26"
equation "\"d38\" = d37"
equation "\"d44\" = 0.5 * d34"
equation "\"d64\" = d34"
equation "\"d78\" = d40"
body "Solid1"
